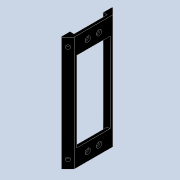
# Autodesk Inventor part: Z Axis Cover Frame
Saved by Autodesk Inventor 2022 (Build 260153000, 153)
## iProperties
Created: 2021-10-26
Part Number: Z Axis Cover Frame
Material: Generic
Document SubType Name: Modeling
Designer: Coy
Density: 1 g/cm^3
Appearance: Anodized - Black
Author: Coy
Autodesk Inventor part; units mm, degrees
ref_plane "YZ Plane" through (0, 0, 0) normal (1, 0, 0) x (0, 1, 0)
ref_plane "XZ Plane" through (0, 0, 0) normal (0, 1, 0) x (-1, 0, 0)
sketch "Sketch1" plane through (0, 0, 0) normal (0, 1, 0) x (-1, 0, 0)
  line L0 (0, 0) -> (0, 68)
  line L1 (0, 0) -> (10.6066, -10.6066)
  line L2 (0, 68) -> (10.6066, 78.6066)
  line L3 (5, 63) -> (5, 5)
  line L4 (10.6066, 78.6066) -> (10.6066, 63)
  line L5 (10.6066, -10.6066) -> (10.6066, 5)
  line L6 (10.6066, 63) -> (5, 63)
  line L7 (10.6066, 5) -> (5, 5)
  line L8 (10.6066, 5) -> (12.1066, 5)
  line L9 (12.1066, 5) -> (12.1066, -10.6066)
  line L10 (12.1066, -10.6066) -> (10.6066, -10.6066)
  line L11 (10.6066, -10.6066) -> (10.6066, 5)
  line L12 (10.6066, 63) -> (12.1066, 63)
  line L13 (12.1066, 63) -> (12.1066, 78.6066)
  line L14 (12.1066, 78.6066) -> (10.6066, 78.6066)
  line L15 (10.6066, 78.6066) -> (10.6066, 63)
  dimension "d0" = 68
  dimension "d1" = 15
  dimension "d2" = 135
  dimension "d4" = 15
  dimension "d5" = 135
  dimension "d6" = 5
  dimension "d7" = 5
  dimension "d8" = 5
  dimension "d35" = 1.5
  constraints: 32 end point, 4 parallel, 4 perpendicular, 3 vertical, 2 horizontal, 1 point on line
  measures "d0" distance of L0.start L0.end
  measures "d1" distance of L0.start L1.end
  measures "d2" angle of L0 L1
  measures "d4" distance of L0.end L2.end
  measures "d5" angle of L0 L2
  measures "d6" distance between parallel lines of L0 L3
  measures "d7" vertical distance of L0.end L4.end
  measures "d8" vertical distance of L0.start L5.end
  measures "d35" distance of L9.end L10.end
extrude "Extrusion1" add sketch "Sketch1" along normal blind 200
sketch "Sketch2" plane through (0, 0, 68) normal (0.7071, 0, 0.7071) x (0.7071, 0, -0.7071)
  line L0 (-15, 0) -> (0, 0) construction
  line L1 (-7.5, 0) -> (-7.5, 200) construction
  circle A0 centre (-7.5, 185) radius 3.45
  circle A1 centre (-7.5, 15) radius 3.45
  line L2 (-15, 200) -> (0, 200) projected
  point P0 (48.0833, 0)
  dimension "d11" = 6.9
  dimension "d12" = 6.9
  dimension "d13" = 15
  dimension "d14" = 15
  constraints: 2 centre point, 2 end point, 2 point on line, 1 midpoint, 1 vertical
  measures "d11" diameter of A0
  measures "d12" diameter of A1
  measures "d13" distance from line of L2 A0.centre
  measures "d14" distance from line of L0 A1.centre
extrude "Extrusion2" cut sketch "Sketch2" against normal blind 6
sketch "Sketch3" plane through (0, 0, 68) normal (1, 0, 0) x (0, 0, -1)
  ellipse E0 centre (-5.3033, 185) end of major axis (-5.3033, 181.55) minor radius 2.4395 construction
  ellipse E1 centre (73.3033, 185) end of major axis (73.3033, 188.45) minor radius 2.4395 construction
  line L0 (-5.3033, 185) -> (73.3033, 185) construction
  ellipse E2 centre (-5.3033, 15) end of major axis (-5.3033, 11.55) minor radius 2.4395 construction
  ellipse E3 centre (73.3033, 15) end of major axis (73.3033, 18.45) minor radius 2.4395 construction
  line L1 (-5.3033, 15) -> (73.3033, 15) construction
  line L2 (0, 200) -> (68, 200) construction
  line L3 (34, 200) -> (34, 0) construction
  line L4 (63, 0) -> (5, 0) construction
  line L5 (44, 200) -> (44, 0) construction
  line L6 (24, 200) -> (24, 0) construction
  circle A0 centre (44, 185) radius 2.6
  circle A1 centre (24, 185) radius 2.6
  circle A2 centre (24, 15) radius 2.6
  circle A3 centre (44, 15) radius 2.6
  point P0 (68, 0)
  dimension "d17" = 10
  dimension "d18" = 10
  dimension "d19" = 5.2
  dimension "d20" = 5.2
  dimension "d21" = 5.2
  dimension "d22" = 5.2
  constraints: 10 end point, 8 point on line, 4 centre point, 2 horizontal, 2 midpoint, 2 parallel, 4 other
  measures "d17" distance between parallel lines of L3 L5
  measures "d18" distance between parallel lines of L3 L6
  measures "d19" diameter of A0
  measures "d20" diameter of A1
  measures "d21" diameter of A2
  measures "d22" diameter of A3
extrude "Extrusion3" cut sketch "Sketch3" against normal up to next
sketch "Sketch4" plane through (0, 0, 68) normal (1, 0, 0) x (0, 0, -1)
  line L0 (5, 0) -> (5, 200) projected
  line L1 (63, 0) -> (63, 200) projected
  line L2 (5, 170) -> (63, 170)
  line L3 (5, 30) -> (63, 30)
  circle A0 centre (24, 185) radius 2.6 projected
  circle A1 centre (24, 15) radius 2.6 projected
  point P0 (68, 0)
  dimension "d25" = 15
  dimension "d26" = 15
  constraints: 4 end point, 4 point on line, 2 perpendicular
  measures "d25" distance from line of A0.centre L2
  measures "d26" distance from line of A1.centre L3
extrude "Extrusion4" cut sketch "Sketch4" against normal up to next contours L0 L2 L1 L3
sketch "Sketch5" plane through (0, 0, 68) normal (1, 0, 0) x (0, 0, -1)
  circle A0 centre (24, 185) radius 2.6 projected
  circle A1 centre (24, 185) radius 4.75
  circle A2 centre (44, 185) radius 2.6 projected
  circle A3 centre (44, 185) radius 4.75
  circle A4 centre (24, 15) radius 2.6 projected
  circle A5 centre (24, 15) radius 4.75
  circle A6 centre (44, 15) radius 2.6 projected
  circle A7 centre (44, 15) radius 4.75
  point P0 (68, 0)
  dimension "d29" = 9.5
  dimension "d30" = 9.5
  dimension "d31" = 9.5
  dimension "d32" = 9.5
  constraints: 4 centre point, 4 coincident
  measures "d29" diameter of A1
  measures "d30" diameter of A3
  measures "d31" diameter of A5
  measures "d32" diameter of A7
extrude "Extrusion5" cut sketch "Sketch5" against normal blind 3
ref_plane "Work Plane2" through (-12.1066, 0, 34) normal (0, 0, 1) x (1, 0, 0)
mirror "Mirror2" about plane through (-12.1066, 0, 34) normal (0, 0, 1) of "Extrusion2"
equation "\"d4\" = d1"
equation "\"d5\" = d2"
equation "\"d12\" = d11"
equation "\"d14\" = d13"
equation "\"d20\" = d19"
equation "\"d21\" = d19"
equation "\"d22\" = d19"
equation "\"d30\" = d29"
equation "\"d31\" = d29"
equation "\"d32\" = d29"
body "Solid1"
